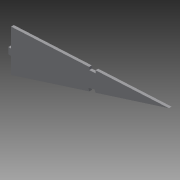
# Autodesk Inventor part: Star Side
Saved by Autodesk Inventor 2015 (Build 190159000, 159)
## iProperties
Created: 2018-03-07
Part Number: Star Side
Material: Generic
Document SubType Name: Modeling
Designer: Administrator
Density: 1 g/cm^3
Appearance: Default
Author: Administrator
Autodesk Inventor part; units mm, degrees
ref_plane "YZ Plane" through (0, 0, 0) normal (1, 0, 0) x (0, 1, 0)
ref_plane "XZ Plane" through (0, 0, 0) normal (0, 1, 0) x (-1, 0, 0)
ref_plane "XY Plane" through (0, 0, 0) normal (0, 0, 1) x (1, 0, 0)
sketch "Sketch1" plane through (0, 0, 0) normal (0, 0, 1) x (1, 0, 0)
  line L0 (0, 0) -> (0, 49.7586)
  line L1 (0, 49.7586) -> (187.6422, 59.5597)
  line L2 (187.6422, 59.5597) -> (0, 0)
  dimension "d0" = 49.7586
  dimension "d40" = 92.99
  dimension "d41" = 72.39
  constraints: 6 end point, 1 vertical
  measures "d0" distance of L0.start L0.end
  measures "d40" angle of L0 L1
  measures "d41" angle of L2 L0
extrude "Extrusion1" add sketch "Sketch1" along normal blind 3.175
sketch "Sketch3" plane through (0, 0, 3.175) normal (0, 0, 1) x (1, 0, 0)
  line L0 (0, 49.7586) -> (0, 0) projected
  line L1 (0, 27.1018) -> (-3.175, 27.1018)
  line L2 (-3.175, 27.1018) -> (-3.175, 19.4818)
  line L3 (-3.175, 19.4818) -> (0, 19.4818)
  line L4 (0, 27.1018) -> (0, 19.4818)
  point P0 (0, 23.2918)
  dimension "d9" = 7.62
  dimension "d11" = 3.175
  dimension "d43" = 26.4668
  dimension "d44" = 3.81
  constraints: 8 end point, 2 perpendicular, 2 point on line, 1 collinear, 1 horizontal, 1 midpoint
  measures "d9" distance of L1.end L2.end
  measures "d11" distance between parallel lines of L0 L2
  measures "d43" distance of L0.start point (0, 23.292)
  measures "d44" distance from line of L3 point (0, 23.292)
extrude "Extrusion3" add sketch "Sketch3" against normal blind 3.175
sketch "Sketch5" plane through (0, 0, 3.175) normal (0, 0, 1) x (1, 0, 0)
  line L0 (187.6422, 59.5597) -> (0, 49.7586) projected
  line L1 (0, 0) -> (187.6422, 59.5597) projected
  line L2 (92.766, 54.604) -> (92.9316, 51.4333)
  line L3 (92.9316, 51.4333) -> (100.5412, 51.8308)
  line L4 (100.5412, 51.8308) -> (100.3756, 55.0015)
  line L5 (92.766, 54.604) -> (100.3756, 55.0015)
  line L6 (100.2023, 31.8053) -> (99.2417, 34.8315)
  line L7 (99.2417, 34.8315) -> (91.9788, 32.5262)
  line L8 (91.9788, 32.5262) -> (92.9393, 29.5)
  line L9 (92.9393, 29.5) -> (100.2023, 31.8053)
  point P0 (96.5708, 54.8028)
  point P1 (96.5708, 30.6526)
  dimension "d32" = 7.62
  dimension "d34" = 3.175
  dimension "d35" = 3.175
  dimension "d36" = 7.62
  dimension "d45" = 96.5708
  dimension "d46" = 96.5708
  dimension "d47" = 3.81
  dimension "d48" = 3.81
  constraints: 16 end point, 6 point on line, 4 parallel, 3 perpendicular, 2 collinear
  measures "d32" distance between parallel lines of L4 L2
  measures "d34" distance between parallel lines of L0 L3
  measures "d35" distance between parallel lines of L1 L7
  measures "d36" distance between parallel lines of L8 L6
  measures "d45" horizontal distance of point (96.571, 54.803) L0.end
  measures "d46" horizontal distance of L1.start point (96.571, 30.653)
  measures "d47" distance from line of L8 point (96.571, 30.653)
  measures "d48" distance from line of L4 point (96.571, 54.803)
extrude "Extrusion5" cut sketch "Sketch5" against normal blind 25.4
sketch "Sketch6" plane through (0, 0, 3.175) normal (0, 0, 1) x (1, 0, 0)
  line L0 (0, 0) -> (0, 19.4818)
  line L1 (0, 19.4818) -> (0, 0) projected
  line L2 (0, 19.4818) -> (-3.175, 19.4818)
  line L3 (-3.175, 19.4818) -> (0, 19.4818) projected
  line L4 (-3.175, 19.4818) -> (-3.175, 27.1018)
  line L5 (-3.175, 27.1018) -> (-3.175, 19.4818) projected
  line L6 (-3.175, 27.1018) -> (0, 27.1018)
  line L7 (0, 27.1018) -> (-3.175, 27.1018) projected
  line L8 (0, 27.1018) -> (0, 49.7586)
  line L9 (0, 49.7586) -> (0, 27.1018) projected
  line L10 (0, 49.7586) -> (92.766, 54.604)
  line L11 (92.766, 54.604) -> (0, 49.7586) projected
  line L12 (92.766, 54.604) -> (92.9316, 51.4333)
  line L13 (92.9316, 51.4333) -> (100.5412, 51.8308)
  line L14 (100.5412, 51.8308) -> (92.9316, 51.4333) projected
  line L15 (100.5412, 51.8308) -> (100.3756, 55.0015)
  line L16 (100.3756, 55.0015) -> (100.5412, 51.8308) projected
  line L17 (100.3756, 55.0015) -> (187.6422, 59.5597)
  line L18 (100.3756, 55.0015) -> (187.6422, 59.5597) projected
  line L19 (187.6422, 59.5597) -> (100.2023, 31.8053)
  line L20 (100.2023, 31.8053) -> (187.6422, 59.5597) projected
  line L21 (100.2023, 31.8053) -> (99.2417, 34.8315)
  line L22 (99.2417, 34.8315) -> (91.9788, 32.5262)
  line L23 (91.9788, 32.5262) -> (92.9393, 29.5)
  line L24 (91.9788, 32.5262) -> (92.9393, 29.5) projected
  line L25 (92.9393, 29.5) -> (0, 0)
  constraints: 30 end point, 11 collinear, 4 perpendicular
body "Solid1"
